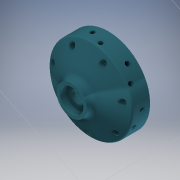
# Autodesk Inventor part: Drum
Saved by Autodesk Inventor 2018 (Build 220112000, 112)
## iProperties
Created: 2023-03-11
Part Number: Drum
Material: Generic
Document SubType Name: Modeling
Designer: Habib Mohamed
Density: 1 g/cm^3
Appearance: Galvanized
Author: Habib Mohamed
Autodesk Inventor part; units mm, degrees
ref_plane "YZ Plane" through (0, 0, 0) normal (1, 0, 0) x (0, 1, 0)
ref_plane "XZ Plane" through (0, 0, 0) normal (0, 1, 0) x (-1, 0, 0)
ref_plane "XY Plane" through (0, 0, 0) normal (0, 0, 1) x (1, 0, 0)
sketch "Sketch1" plane through (0, 0, 0) normal (1, 0, 0) x (0, 1, 0)
  line L0 (0, 60.4181) -> (0, -60.4181) construction
  line L1 (14, 0) -> (14, -8)
  line L2 (14, -8) -> (8, -8)
  line L3 (8, -8) -> (8, -11.5)
  line L4 (8, -11.5) -> (19.1801, -11.5)
  line L5 (19.1801, -11.5) -> (36.0783, -19.9509)
  line L6 (40.5, -27.1061) -> (40.5, -38)
  line L7 (40.5, -38) -> (45, -38)
  line L8 (45, -38) -> (45, -44)
  line L9 (45, -44) -> (50, -44)
  line L10 (50, -44) -> (50, -24.8539)
  line L11 (48.3419, -22.1708) -> (22.4217, -9.2079)
  line L12 (18, -2.0528) -> (18, 0)
  line L13 (18, 0) -> (14, 0)
  arc A0 (18, -2.0528) -> (22.4217, -9.2079) centre (26, -2.0528) ccw
  arc A1 (50, -24.8539) -> (48.3419, -22.1708) centre (47, -24.8539) ccw
  arc A2 (40.5, -27.1061) -> (36.0783, -19.9509) centre (32.5, -27.1061) ccw
  line L14 (42.3074, -19.1529) -> (50, -23) construction
  line L15 (50, -11.2983) -> (50, -23) construction
  line L16 (18, -2.0528) -> (18, -6.9965) construction
  line L17 (18, -6.9965) -> (22.4217, -9.2079) construction
  point P0 (0, 0)
  point P1 (0, 0)
  dimension "d0" = 50
  dimension "d1" = 45
  dimension "d2" = 40.5
  dimension "d3" = 6
  dimension "d4" = 32.5
  dimension "d5" = 44
  dimension "d6" = 3.5
  dimension "d7" = 18
  dimension "d8" = 14
  dimension "d9" = 26.57
  dimension "d10" = 8
  dimension "d11" = 3.5
  dimension "d12" = 8
  dimension "d13" = 3
  dimension "d37" = 21
  constraints: 36 end point, 8 perpendicular, 6 point on circle, 6 tangent, 4 collinear, 3 centre point, 3 parallel, 3 vertical, 1 coincident, 1 equal radius, 1 midpoint, 1 point on line
  measures "d0" distance between parallel lines of L0 L10
  measures "d1" distance between parallel lines of L0 L8
  measures "d2" distance between parallel lines of L0 L6
  measures "d3" distance of L7.end L8.end
  measures "d4" distance between parallel lines of L4 L9
  measures "d5" distance between parallel lines of L9 L13
  measures "d6" distance between parallel lines of L11 L5
  measures "d7" distance between parallel lines of L12 L0
  measures "d8" distance between parallel lines of L0 L1
  measures "d9" angle of L9 L5
  measures "d10" distance between parallel lines of L0 L3
  measures "d11" distance between parallel lines of L2 L4
  measures "d12" radius of A0
  measures "d13" radius of A1
  measures "d37" distance from line of L9 L14.end
revolve "Revolution1" add sketch "Sketch1" angle 360 about axis through (0, 0, 60.4181) along (0, 0, -1)
sketch "Sketch2" plane through (0, 0, 0) normal (0, 1, 0) x (-1, 0, 0)
  circle A0 centre (9, -34) radius 2.5
  circle A1 centre (-7, -27.5) radius 2.5
  line L0 (0, -9.8686) -> (0, -47.9738) construction
  line L1 (-50, -44) -> (50, -44) projected
  point P0 (0, 0)
  dimension "d15" = 5
  dimension "d16" = 7
  dimension "d17" = 9
  dimension "d18" = 10
  dimension "d19" = 16.5
  constraints: 2 centre point, 2 end point, 1 equal radius, 1 point on line, 1 vertical
  measures "d15" diameter of A0
  measures "d16" distance from line of L0 A1.centre
  measures "d17" distance from line of L0 A0.centre
  measures "d18" distance from line of A0.centre L1
  measures "d19" distance from line of A1.centre L1
extrude "Extrusion1" cut sketch "Sketch2" along normal blind 59.5
sketch "Sketch3" plane through (0, 0, -38) normal (0, 0, -1) x (-1, 0, 0)
  arc A0 (-9.4688, 39.3776) -> (-4.5312, 40.2457) centre (0, 0) ccw construction
  point P0 (0, 0)
  point P1 (0, -42.5)
  point P2 (0, -42.5)
  dimension "d38" = 42.5
  constraints: 1 coincident, 1 vertical alignment
  measures "d38" distance of point (0, -42.5) point (0, 0)
hole "Hole1" at (0, -42.5, -38) direction (0, 0, 1) diameter 4 depth 24.5
sketch "Sketch4" plane through (0, 0, 0) normal (1, 0, 0) x (0, 1, 0)
  line L0 (-45, -38) -> (45, -38) construction
  line L1 (-42.5, -38) -> (-42.5, 4.9936) construction
  line L2 (-42.5, -21.5) -> (-39, -21.5)
  line L3 (-39, -21.5) -> (-39, -16.5)
  line L4 (-39, -16.5) -> (-42.5, -16.5)
  line L5 (-42.5, -16.5) -> (-42.5, -21.5)
  line L6 (-40.5, -18.249) -> (-40.5, -38) construction
  line L7 (-40.5, -38) -> (-44.5, -38) construction
  line L8 (-44.5, -20.2494) -> (-44.5, -38) construction
  line L9 (-45, -44) -> (45, -44) projected
  point P0 (0, 0)
  dimension "d30" = 3.5
  dimension "d32" = 5
  dimension "d42" = 22.5
  constraints: 12 end point, 7 point on line, 2 parallel, 1 horizontal, 1 midpoint, 1 perpendicular, 1 vertical
  measures "d30" distance of L3.end L4.end
  measures "d32" distance of L2.end L3.end
  measures "d42" distance between parallel lines of L9 L2
revolve "Revolution2" cut sketch "Sketch4" angle 360 about axis through (0, -42.5, -38) along (0, 0, 1)
sketch "Sketch5" plane through (0, 0, -38) normal (0, 0, -1) x (-1, 0, 0)
  circle A0 centre (0, -42.5) radius 2 projected
  circle A1 centre (0, -42.5) radius 2.5
  circle A2 centre (0, 0) radius 36.0783 construction
  circle A3 centre (0, 0) radius 19.1801 construction
  point P0 (0, 0)
  point P1 (0, -40.5)
  dimension "d39" = 5
  constraints: 1 centre point, 1 coincident, 1 vertical alignment
  measures "d39" diameter of A1
extrude "Extrusion2" add sketch "Sketch5" against normal through all
pattern_circular "Circular Pattern1" count 7 over 360 about axis through (0, 0, -34.427) along (0, 0, -1) of "Extrusion1", "Hole1", "Revolution2", "Extrusion2"
equation "\"d11\" = d6"
body "Solid1"
